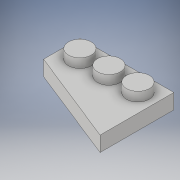
# Autodesk Inventor part: other diagonal piece
Saved by Autodesk Inventor 2017 (Build 210142000, 142)
## iProperties
Created: 2018-05-17
Part Number: other diagonal piece
Material: Generic
Document SubType Name: Modeling
Designer: 20000650
Density: 1 g/cm^3
Appearance: Default
Author: 20000650
Autodesk Inventor part; units mm, degrees
ref_plane "YZ Plane" through (0, 0, 0) normal (1, 0, 0) x (0, 1, 0)
ref_plane "XZ Plane" through (0, 0, 0) normal (0, 1, 0) x (-1, 0, 0)
ref_plane "XY Plane" through (0, 0, 0) normal (0, 0, 1) x (1, 0, 0)
sketch "Sketch1" plane through (0, 0, 0) normal (0, 1, 0) x (-1, 0, 0)
  line L0 (0, 0) -> (0, 15.8369)
  line L1 (0, 0) -> (20.1574, 0)
  line L2 (20.1574, 0) -> (20.1574, 7.7978)
  line L3 (20.1574, 7.7978) -> (0, 15.8369)
  dimension "d0" = 15.8369
  dimension "d1" = 20.1574
  dimension "d2" = 7.7978
  constraints: 8 end point, 2 vertical, 1 horizontal
  measures "d0" distance of L0.start L0.end
  measures "d1" distance of L0.start L1.end
  measures "d2" distance of L1.end L2.end
extrude "Extrusion1" add sketch "Sketch1" along normal blind 3.236
sketch "Sketch2" plane through (0, 3.236, 0) normal (0, 1, 0) x (1, 0, 0)
  line L0 (-20.1574, -7.7978) -> (0, -15.8369) projected
  line L1 (-20.1574, 0) -> (-20.1574, -7.7978)
  line L2 (0, 0) -> (-20.1574, 0) projected
  line L3 (-20.1574, 0) -> (-20.1574, -7.7978)
  circle A0 centre (-16.2585, -3.8989) radius 2.4498
  dimension "d7" = 4.8997
  constraints: 4 end point, 1 centre point
  measures "d7" diameter of A0
extrude "Extrusion2" add sketch "Sketch2" along normal blind 1.9837
pattern_linear "Rectangular Pattern1" count 3 spacing 6.223 along (1, 0, 0) of "Extrusion2"
body "Solid1"
